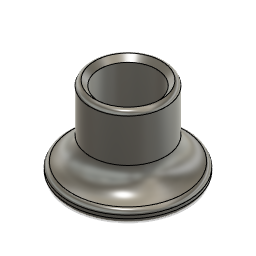
Landing feet v1 (Autodesk Fusion 360 design; units mm, degrees)
Autodesk Fusion 360 part; units mm, degrees
sketch "Sketch1" plane through (0, 0, 0) normal (0, 1, 0) x (1, 0, 0)
  circle A0 centre (0, 0) radius 12.5
  dimension "d1" = 25
  constraint coincident A0.centre origin
  measures "d1" diameter of A0
extrude "Extrude1" add sketch "Sketch1" along normal blind 2.5
sketch "Sketch2" plane through (0, 2.5, 0) normal (0, 1, 0) x (-1, 0, 0)
  circle A0 centre (0, 0) radius 12.5
  circle A1 centre (0, 0) radius 7.9
  circle A2 centre (0, 0) radius 6
  dimension "d4" = 15.8
  dimension "d5" = 12
  constraint concentric A0 A1
  constraint concentric A0 A2
  measures "d4" diameter of A1
  measures "d5" diameter of A2
extrude "Extrude2" add sketch "Sketch2" along normal blind 15 contours A1
fillet "Fillet1" radius 5 1 edges at (7.3654, 2.5, 2.8568)
fillet "Fillet2" radius 1 2 edges at (-11.6541, 2.5, 4.5202) (-11.6541, 0, 4.5202)
chamfer "Chamfer1" distance 1 angle 45 1 edges at (5.594, 17.5, 2.1697)
fillet "Fillet3" radius 1 1 edges at (7.3654, 17.5, -2.8568)
